Autodesk Fusion 360 part; units mm, degrees
note: some values were not read from the file. Set by a fixed rule: which face or edge a step refers to.
(part 2 of 5)
sketch "Sketch25" plane through (0, 0, 115) normal (0, 0, 1) x (-1, 0, 0)
  line L0 (-26, -108.2203) -> (-26, -178)
  line L1 (-26, -178) -> (-184, -178)
  line L2 (-184, -178) -> (-184, -108.2203)
  line L3 (-184, -108.2203) -> (-180.316, -106.8794)
  arc A0 (-180.316, -106.8794) -> (-179, -105) centre (-181, -105) ccw
  line L4 (-179, -105) -> (-179, -99)
  arc A1 (-179, -99) -> (-180.316, -97.1206) centre (-181, -99) ccw
  line L5 (-180.316, -97.1206) -> (-184, -95.7797)
  line L6 (-184, -95.7797) -> (-184, -56)
  spline S0 degree 3 poles (-184, -56) (-184, -53.3075) (-183.9037, -51.0109) (-183.6552, -49.1696) (-183.4152, -47.3913) (-183.0542, -46.0543) (-182.4179, -44.7239) (-181.7989, -43.4297) (-180.8711, -42.0696) (-179.3518, -40.4458) (-177.5325, -38.5013) (-174.8564, -36.2157) (-171.5158, -33.7703) (-166.6133, -30.1816) (-160.3099, -26.2473) (-154.1768, -22.9953) (-150.0182, -20.7903) (-145.9518, -18.9172) (-142.5291, -17.6934) (-139.736, -16.6948) (-137.3746, -16.1501) (-135.7618, -16.0299) (-135.486, -16.0093) (-135.2319, -16) (-135, -16) knots -1 -1 -1 -1 -0.872949 -0.872949 -0.872949 -0.750244 -0.750244 -0.750244 -0.630875 -0.630875 -0.630875 -0.48793 -0.48793 -0.48793 -0.278155 -0.278155 -0.278155 -0.135918 -0.135918 -0.135918 -0.019847 -0.019847 -0.019847 0 0 0 0
  line L7 (-135, -16) -> (-75, -16)
  spline S1 degree 3 poles (-75, -16) (-73.6407, -16) (-71.4915, -16.3704) (-68.8469, -17.2246) (-63.8244, -18.8468) (-57.0667, -22.1371) (-50.6302, -25.8861) (-45.8029, -28.6979) (-41.1682, -31.7394) (-37.4534, -34.5352) (-34.6662, -36.633) (-32.4058, -38.5922) (-30.788, -40.2974) (-29.2773, -41.8897) (-28.3285, -43.2367) (-27.6926, -44.499) (-27.0341, -45.806) (-26.6597, -47.0839) (-26.4026, -48.7672) (-26.1107, -50.6784) (-26, -53.108) (-26, -56) knots 0 0 0 0 0.116327 0.116327 0.116327 0.337245 0.337245 0.337245 0.502934 0.502934 0.502934 0.627254 0.627254 0.627254 0.743338 0.743338 0.743338 0.863534 0.863534 0.863534 1 1 1 1
  line L8 (-26, -56) -> (-26, -95.7797)
  line L9 (-26, -95.7797) -> (-29.684, -97.1206)
  arc A2 (-29.684, -97.1206) -> (-31, -99) centre (-29, -99) ccw
  line L10 (-31, -99) -> (-31, -105)
  line L11 (-26, -104.5) -> (-28.6, -104.5)
  line L12 (-28.6, -104.5) -> (-28.6, -102)
  line L13 (-29.5, -99.2) -> (-26, -99.2)
  line L14 (-184, -99.2) -> (-180.5, -99.2)
  line L15 (-180.5, -99.2) -> (-180.5, -104.8)
  line L16 (-180.5, -104.8) -> (-184, -104.8)
  line L17 (-30, 0) -> (-180, 0)
  arc A3 (-180, 0) -> (-210, -30) centre (-180, -30) ccw
  line L18 (-210, -30) -> (-210, -180)
  arc A4 (-210, -180) -> (-180, -210) centre (-180, -180) ccw
  line L19 (-180, -210) -> (-30, -210)
  arc A5 (-30, -210) -> (0, -180) centre (-30, -180) ccw
  line L20 (0, -180) -> (0, -30)
  arc A6 (0, -30) -> (-30, 0) centre (-30, -30) ccw
  line L21 (-31, -102) -> (-31, -178)
  line L22 (-31, -102) -> (-31, -30)
  line L23 (-179, -102) -> (-179, -178)
  line L24 (-179, -102) -> (-179, -26)
  line L25 (-26, -99.2) -> (-26, -104.5)
  arc A7 (-31, -105) -> (-29.684, -106.8794) centre (-29, -105) ccw
  line L26 (-29.684, -106.8794) -> (-26, -108.2203)
  circle A8 centre (-199, -108) radius 3.5
  circle A9 centre (-11, -108) radius 3.5
  ellipse E0 centre (-105, -188.2858) end of major axis (-105, -180.5592) minor radius 5.4567
  circle A10 centre (-199, -175) radius 2
  circle A11 centre (-199, -35) radius 2
  circle A12 centre (-11, -35) radius 2
  line L27 (-28.6, -102) -> (-29.5, -102)
  line L28 (-29.5, -102) -> (-29.5, -99.2)
  line L29 (-184, -104.8) -> (-184, -99.2)
  circle A13 centre (-11, -70) radius 2
  circle A14 centre (-199, -70) radius 2
  circle A15 centre (-11, -140) radius 2
  circle A16 centre (-11, -175) radius 2
  circle A17 centre (-199, -140) radius 2
  constraint midpoint L10 L21.start
  constraint coincident L1 L21.end
  constraint perpendicular L1 L21
  constraint parallel L10 L22
  constraint midpoint L4 L23.start
  constraint coincident L1 L23.end
  constraint perpendicular L1 L23
  constraint parallel L4 L24
extrude "Extrude1'" add sketch "Sketch25" along normal blind 10 separate body contours L0 L1 L21 A7 L26 | L1 L2 L3 A0 L23 | S1 L8 L9 A2 L22 | A1 L5 L6 S0 L24 | L11 L12 L13 L25 L27 L28 | L14 L15 L16 L29 | L17 A3 L18 A4 L19 A5 L20 A6 | A8 | A9 makes body 5 in component "inner_adapter"
sketch "Sketch33" plane through (0, 0, 125) normal (0, 0, 1) x (-1, 0, 0)
  line L0 (-179, -178) -> (-179, -40.0766)
  spline S0 degree 3 poles (-179, -40.0766) (-177.1947, -38.2144) (-174.6472, -36.0625) (-171.5158, -33.7703) (-166.6133, -30.1816) (-160.3099, -26.2473) (-154.1768, -22.9953) (-150.0182, -20.7903) (-145.9518, -18.9172) (-142.5291, -17.6934) (-139.736, -16.6948) (-137.3746, -16.1501) (-135.7618, -16.0299) (-135.486, -16.0093) (-135.2319, -16) (-135, -16) knots -0.621923 -0.621923 -0.621923 -0.621923 -0.48793 -0.48793 -0.48793 -0.278155 -0.278155 -0.278155 -0.135918 -0.135918 -0.135918 -0.019847 -0.019847 -0.019847 0 0 0 0
  line L1 (-135, -16) -> (-75, -16)
  spline S1 degree 3 poles (-75, -16) (-73.6407, -16) (-71.4915, -16.3704) (-68.8469, -17.2246) (-63.8244, -18.8468) (-57.0667, -22.1371) (-50.6302, -25.8861) (-45.8029, -28.6979) (-41.1682, -31.7394) (-37.4534, -34.5352) (-34.7859, -36.5429) (-32.601, -38.4237) (-31, -40.0763) knots 0 0 0 0 0.116327 0.116327 0.116327 0.337245 0.337245 0.337245 0.502934 0.502934 0.502934 0.621914 0.621914 0.621914 0.621914
  line L2 (-31, -40.0763) -> (-31, -178)
  line L3 (-31, -178) -> (-179, -178)
  arc A0 (0, -30) -> (-30, 0) centre (-30, -30) ccw
  line L4 (-30, 0) -> (-180, 0)
  arc A1 (-180, 0) -> (-210, -30) centre (-180, -30) ccw
  line L5 (-210, -30) -> (-210, -180)
  arc A2 (-210, -180) -> (-180, -210) centre (-180, -180) ccw
  line L6 (-180, -210) -> (-30, -210)
  arc A3 (-30, -210) -> (0, -180) centre (-30, -180) ccw
  line L7 (0, -180) -> (0, -30)
  line L8 (-109.7559, -178) -> (-100.2441, -178)
  ellipse E0 centre (-105, -188.2858) end of major axis (-105, -180.5592) minor radius 5.4567
  circle A4 centre (-11, -175) radius 2
  circle A5 centre (-199, -175) radius 2
  circle A6 centre (-11, -35) radius 2
  circle A7 centre (-199, -35) radius 2
  circle A8 centre (-199, -35) radius 3.5
  circle A9 centre (-199, -175) radius 3.5
  circle A10 centre (-11, -175) radius 3.5
  circle A11 centre (-11, -35) radius 3.5
  circle A12 centre (-11, -35) radius 2
  ellipse E1 centre (-105, -188.2858) end of major axis (-105, -180.5592) minor radius 5.4567
  circle A13 centre (-199, -175) radius 2
  circle A14 centre (-199, -35) radius 2
  circle A15 centre (-199, -140) radius 2
  circle A16 centre (-11, -140) radius 2
  circle A17 centre (-199, -70) radius 2
  circle A18 centre (-11, -175) radius 2
  circle A19 centre (-11, -70) radius 2
  dimension "d225" = 7
  dimension "d226" = 7
  dimension "d227" = 7
  dimension "d228" = 7
  constraint concentric A7 A8
  constraint concentric A5 A9
  constraint concentric A4 A10
  constraint concentric A6 A11
  measures "d225" diameter of A8
  measures "d226" diameter of A9
  measures "d227" diameter of A10
  measures "d228" diameter of A11
extrude "Extrude5'" cut sketch "Sketch33" against normal blind 5 contours A8 | A9 | A10 | A11 bodies 5 in component "inner_adapter"
sketch "Sketch34" plane through (0, 0, 125) normal (0, 0, 1) x (-1, 0, 0)
  circle A0 centre (-11, -175) radius 3.5
  circle A1 centre (-199, -175) radius 3.5
  circle A2 centre (-11, -35) radius 3.5
  circle A3 centre (-199, -35) radius 3.5
  line L0 (-179, -178) -> (-179, -40.0766)
  spline S0 degree 3 poles (-179, -40.0766) (-177.1947, -38.2144) (-174.6472, -36.0625) (-171.5158, -33.7703) (-166.6133, -30.1816) (-160.3099, -26.2473) (-154.1768, -22.9953) (-150.0182, -20.7903) (-145.9518, -18.9172) (-142.5291, -17.6934) (-139.736, -16.6948) (-137.3746, -16.1501) (-135.7618, -16.0299) (-135.486, -16.0093) (-135.2319, -16) (-135, -16) knots -0.621923 -0.621923 -0.621923 -0.621923 -0.48793 -0.48793 -0.48793 -0.278155 -0.278155 -0.278155 -0.135918 -0.135918 -0.135918 -0.019847 -0.019847 -0.019847 0 0 0 0
  line L1 (-135, -16) -> (-75, -16)
  spline S1 degree 3 poles (-75, -16) (-73.6407, -16) (-71.4915, -16.3704) (-68.8469, -17.2246) (-63.8244, -18.8468) (-57.0667, -22.1371) (-50.6302, -25.8861) (-45.8029, -28.6979) (-41.1682, -31.7394) (-37.4534, -34.5352) (-34.7859, -36.5429) (-32.601, -38.4237) (-31, -40.0763) knots 0 0 0 0 0.116327 0.116327 0.116327 0.337245 0.337245 0.337245 0.502934 0.502934 0.502934 0.621914 0.621914 0.621914 0.621914
  line L2 (-31, -40.0763) -> (-31, -178)
  line L3 (-31, -178) -> (-179, -178)
  arc A4 (0, -30) -> (-30, 0) centre (-30, -30) ccw
  line L4 (-30, 0) -> (-180, 0)
  arc A5 (-180, 0) -> (-210, -30) centre (-180, -30) ccw
  line L5 (-210, -30) -> (-210, -180)
  arc A6 (-210, -180) -> (-180, -210) centre (-180, -180) ccw
  line L6 (-180, -210) -> (-30, -210)
  arc A7 (-30, -210) -> (0, -180) centre (-30, -180) ccw
  line L7 (0, -180) -> (0, -30)
  circle A8 centre (-11, -175) radius 3.5
  circle A9 centre (-199, -175) radius 3.5
  circle A10 centre (-11, -35) radius 3.5
  circle A11 centre (-199, -35) radius 3.5
  line L8 (-179, -178) -> (-179, -40.0766)
  spline S2 degree 3 poles (-179, -40.0766) (-177.1947, -38.2144) (-174.6472, -36.0625) (-171.5158, -33.7703) (-166.6133, -30.1816) (-160.3099, -26.2473) (-154.1768, -22.9953) (-150.0182, -20.7903) (-145.9518, -18.9172) (-142.5291, -17.6934) (-139.736, -16.6948) (-137.3746, -16.1501) (-135.7618, -16.0299) (-135.486, -16.0093) (-135.2319, -16) (-135, -16) knots -0.621923 -0.621923 -0.621923 -0.621923 -0.48793 -0.48793 -0.48793 -0.278155 -0.278155 -0.278155 -0.135918 -0.135918 -0.135918 -0.019847 -0.019847 -0.019847 0 0 0 0
  line L9 (-135, -16) -> (-75, -16)
  spline S3 degree 3 poles (-75, -16) (-73.6407, -16) (-71.4915, -16.3704) (-68.8469, -17.2246) (-63.8244, -18.8468) (-57.0667, -22.1371) (-50.6302, -25.8861) (-45.8029, -28.6979) (-41.1682, -31.7394) (-37.4534, -34.5352) (-34.7859, -36.5429) (-32.601, -38.4237) (-31, -40.0763) knots 0 0 0 0 0.116327 0.116327 0.116327 0.337245 0.337245 0.337245 0.502934 0.502934 0.502934 0.621914 0.621914 0.621914 0.621914
  line L10 (-31, -40.0763) -> (-31, -178)
  line L11 (-31, -178) -> (-179, -178)
  arc A12 (0, -30) -> (-30, 0) centre (-30, -30) ccw
  line L12 (-30, 0) -> (-180, 0)
  arc A13 (-180, 0) -> (-210, -30) centre (-180, -30) ccw
  line L13 (-210, -30) -> (-210, -180)
  arc A14 (-210, -180) -> (-180, -210) centre (-180, -180) ccw
  line L14 (-180, -210) -> (-30, -210)
  arc A15 (-30, -210) -> (0, -180) centre (-30, -180) ccw
  line L15 (0, -180) -> (0, -30)
  line L16 (-179.0609, -163) -> (-179, -173)
  line L17 (-184, -183) -> (-184, -38.0508)
  spline S4 degree 3 poles (-184, -38.0508) (-183.53, -37.5659) (-183.0599, -37.0811) (-182.5899, -36.5963) (-180.4883, -34.4285) (-177.7611, -32.1455) (-174.4691, -29.7357) (-169.3238, -25.9693) (-162.8741, -21.9475) (-156.519, -18.5779) (-152.2041, -16.29) (-147.9761, -14.3309) (-144.2124, -12.9853) (-141.9329, -12.1703) (-139.8769, -11.6068) (-138.0391, -11.287) (-137.3844, -11.1731) (-136.7557, -11.0901) (-136.1336, -11.0437) (-135.7424, -11.0145) (-135.3658, -11) (-135, -11) knots -0.65681 -0.65681 -0.65681 -0.65681 -0.621923 -0.621923 -0.621923 -0.48793 -0.48793 -0.48793 -0.278155 -0.278155 -0.278155 -0.135918 -0.135918 -0.135918 -0.050335 -0.050335 -0.050335 -0.019847 -0.019847 -0.019847 0 0 0 0
  line L18 (-135, -11) -> (-75, -11)
  spline S5 degree 3 poles (-75, -11) (-73.6669, -11) (-72.3215, -11.1868) (-70.7827, -11.5209) (-69.7039, -11.7551) (-68.5449, -12.0678) (-67.3101, -12.4666) (-63.5716, -13.6741) (-59.3264, -15.5672) (-54.921, -17.8316) (-52.6617, -18.993) (-50.3688, -20.252) (-48.1137, -21.5656) (-43.134, -24.4661) (-38.3659, -27.5905) (-34.4467, -30.5403) (-31.6285, -32.6614) (-29.2725, -34.6734) (-27.4088, -36.5974) (-26.9392, -37.0821) (-26.4696, -37.5669) (-26, -38.0516) knots 0 0 0 0 0.068385 0.068385 0.068385 0.116327 0.116327 0.116327 0.262353 0.262353 0.262353 0.337245 0.337245 0.337245 0.502934 0.502934 0.502934 0.621914 0.621914 0.621914 0.656812 0.656812 0.656812 0.656812
  line L19 (-26, -38.0516) -> (-26, -183)
  line L20 (-26, -183) -> (-184, -183)
  line L21 (-135, -17) -> (-75, -17)
  spline S6 degree 3 poles (-75, -17) (-73.8223, -17) (-71.7285, -17.3447) (-69.1542, -18.1762) (-64.2585, -19.7574) (-57.5268, -23.0263) (-51.1335, -26.7502) (-46.3366, -29.5442) (-41.7286, -32.5691) (-38.0548, -35.3342) (-35.5737, -37.2016) (-33.5233, -38.9532) (-32, -40.4851) knots 0 0 0 0 0.116327 0.116327 0.116327 0.337245 0.337245 0.337245 0.502934 0.502934 0.502934 0.61486 0.61486 0.61486 0.61486
  line L22 (-32, -40.4851) -> (-32, -177)
  line L23 (-32, -177) -> (-178, -177)
  line L24 (-178, -177) -> (-178, -40.4855)
  spline S7 degree 3 poles (-178, -40.4855) (-176.2702, -38.7472) (-173.8613, -36.7265) (-170.9251, -34.5772) (-166.0712, -31.0241) (-159.7971, -27.1072) (-153.7083, -23.8788) (-149.581, -21.6904) (-145.547, -19.8344) (-142.1924, -18.6351) (-139.459, -17.6578) (-137.1491, -17.1361) (-135.6875, -17.0271) (-135.4348, -17.0083) (-135.2051, -17) (-135, -17) knots -0.614871 -0.614871 -0.614871 -0.614871 -0.48793 -0.48793 -0.48793 -0.278155 -0.278155 -0.278155 -0.135918 -0.135918 -0.135918 -0.019847 -0.019847 -0.019847 0 0 0 0
  ellipse E0 centre (-105, -188.2858) end of major axis (-105, -180.5592) minor radius 5.4567
  ellipse E1 centre (-105, -188.2858) end of major axis (-105, -180.5592) minor radius 5.4567
  circle A16 centre (-199, -140) radius 2
  circle A17 centre (-11, -140) radius 2
  circle A18 centre (-199, -70) radius 2
  circle A19 centre (-11, -70) radius 2
  circle A20 centre (-199, -140) radius 2
  circle A21 centre (-11, -140) radius 2
  circle A22 centre (-199, -70) radius 2
  circle A23 centre (-11, -70) radius 2
  dimension "d234" = -5
  dimension "d235" = 1
  constraint coincident L8 L16.end
extrude "Extrude6'" add sketch "Sketch34" along normal blind 80 contours L17 S4 L18 S5 L19 L20 E0 E1 | L20 E0 E1 picked at (-103.7762, -182.6498) bodies 5 in component "inner_adapter"
ref_plane "WorkPlane5" through (184, 102, 115) normal (0.422618, 0, 0.906308) x (0, -1, 0)
sketch "Sketch35" plane through (184, 102, 115) normal (0.422618, 0, 0.906308) x (0, -1, 0)
  line L0 (-2.8, -3.1721) -> (-2.8, 0)
  line L1 (-2.8, -3.1721) -> (2.8, -3.1721)
  line L2 (2.8, -3.1721) -> (2.8, 0)
  line L3 (-2.8, 0) -> (2.8, 0)
extrude "Extrude7" cut sketch "Sketch35" along normal blind 15 and the other way blind 2 bodies 5 in component "inner_adapter"
ref_plane "WorkPlane6" through (105, 109.0383, 160) normal (-1, 0, 0) x (0, -1, 0)
mirror "Mirror1" about plane through (105, 109.0383, 160) normal (-1, 0, 0) of "Extrude7" in component "inner_adapter"
sketch "Sketch36" plane through (179, 0, 0) normal (-1, 0, 0) x (0, -1, 0)
  line L0 (-178, 115) -> (-40.0766, 115)
  line L1 (-40.0766, 115) -> (-40.0766, 205)
  line L2 (-40.0766, 205) -> (-178, 205)
  line L3 (-178, 205) -> (-178, 115)
  circle A0 centre (-173, 130) radius 3.5
  line L4 (-173, 130) -> (-176.5, 130)
  line L5 (-176.5, 130) -> (-176.5, 205)
  line L6 (-176.5, 205) -> (-173, 205)
  line L7 (-173, 130) -> (-169.5, 130)
  line L8 (-169.5, 130) -> (-169.5, 205)
  line L9 (-169.5, 205) -> (-173, 205)
  line L10 (-173, 205) -> (-173, 130)
  line L11 (-171.5, 133.1623) -> (-171.5, 205)
  line L12 (-180, 125) -> (-30, 125)
  dimension "d245" = 7
  dimension "d246" = 5
  dimension "d247" = 3.5
  dimension "d248" = 3.5
  dimension "d267" = 5
  dimension "d412" = 5
  constraint horizontal L4
  constraint vertical L5
  constraint horizontal L6
  constraint coincident L2 L5.end
  constraint coincident A0.centre L4.start
  constraint horizontal L7
  constraint vertical L8
  constraint horizontal L9
  constraint vertical L10
  constraint coincident L2 L8.end
  constraint coincident A0 L11.start
  constraint coincident L2 L11.end
  constraint perpendicular L2 L11
  measures "d245" diameter of A0
  measures "d246" distance of L3 A0.centre
  measures "d247" distance of A0.centre L4.end
  measures "d248" distance of A0.centre L7.end
  measures "d267" distance of L5 L11
  measures "d412" distance of L4 L12
extrude "Extrude8'" cut sketch "Sketch36" against normal blind 5 contours L2 A0 L5 L6 L10 | L2 A0 L9 L10 L11 | A0 L4 L7 | A0 L4 L10 | A0 L7 L10 bodies 5 in component "inner_adapter"
mirror "Mirror2" about plane through (105, 109.0383, 160) normal (-1, 0, 0) of "Extrude8'" in component "inner_adapter"
ref_plane "WorkPlane7" through (180.7273, 173, 126.5) normal (0, 0, 1) x (0, 1, 0)
sketch "Sketch38" plane through (180.1788, 173, 126.5) normal (0, 0, 1) x (1, 0, 0)
  line L0 (-1.1788, 3.5) -> (3.8212, 3.5)
  line L1 (-1.1788, 3) -> (3.8212, 3)
  line L2 (-1.1788, 3) -> (-2.1788, 3)
  spline S0 degree 3 poles (-1.1788, -132.9234) (-2.9841, -134.7856) (-5.5316, -136.9375) (-8.663, -139.2297) (-13.5655, -142.8184) (-19.8689, -146.7527) (-26.0021, -150.0047) (-30.1606, -152.2097) (-34.227, -154.0828) (-37.6497, -155.3066) (-40.4428, -156.3052) (-42.8042, -156.8499) (-44.417, -156.9701) (-44.6928, -156.9907) (-44.9469, -157) (-45.1788, -157) knots -0.621923 -0.621923 -0.621923 -0.621923 -0.48793 -0.48793 -0.48793 -0.278155 -0.278155 -0.278155 -0.135918 -0.135918 -0.135918 -0.019847 -0.019847 -0.019847 0 0 0 0
  line L3 (-45.1788, -157) -> (-105.1788, -157)
  spline S1 degree 3 poles (-105.1788, -157) (-106.5381, -157) (-108.6873, -156.6296) (-111.332, -155.7754) (-116.3544, -154.1532) (-123.1121, -150.8629) (-129.5486, -147.1139) (-134.376, -144.3021) (-139.0107, -141.2606) (-142.7254, -138.4648) (-145.3929, -136.4571) (-147.5779, -134.5763) (-149.1788, -132.9237) knots 0 0 0 0 0.116327 0.116327 0.116327 0.337245 0.337245 0.337245 0.502934 0.502934 0.502934 0.621914 0.621914 0.621914 0.621914
  line L4 (3.8212, -1.4285) -> (3.8212, 3)
  line L5 (-149.1788, -132.9237) -> (-149.1788, -1.5)
  line L6 (-1.1788, -1.5) -> (-1.1788, -132.9234)
  line L7 (-1.1788, 5) -> (-1.1788, 3.5)
  line L8 (3.8212, 3.5) -> (3.8212, -3.5)
  line L9 (-2.1774, 2.972) -> (-2.1774, 3.972)
  line L10 (-2.1788, -1.5) -> (-2.1788, -132.5145)
  spline S2 degree 3 poles (-2.1788, -132.5145) (-3.9086, -134.2528) (-6.3175, -136.2735) (-9.2537, -138.4228) (-14.1076, -141.9759) (-20.3818, -145.8928) (-26.4705, -149.1212) (-30.5978, -151.3096) (-34.6319, -153.1656) (-37.9864, -154.3649) (-40.7198, -155.3422) (-43.0297, -155.8639) (-44.4914, -155.9729) (-44.7441, -155.9917) (-44.9737, -156) (-45.1788, -156) knots -0.614871 -0.614871 -0.614871 -0.614871 -0.48793 -0.48793 -0.48793 -0.278155 -0.278155 -0.278155 -0.135918 -0.135918 -0.135918 -0.019847 -0.019847 -0.019847 0 0 0 0
  line L11 (-45.1788, -156) -> (-105.1788, -156)
  spline S3 degree 3 poles (-105.1788, -156) (-106.3565, -156) (-108.4503, -155.6553) (-111.0246, -154.8238) (-115.9203, -153.2426) (-122.652, -149.9737) (-129.0453, -146.2498) (-133.8422, -143.4558) (-138.4502, -140.4309) (-142.1241, -137.6658) (-144.6051, -135.7984) (-146.6556, -134.0468) (-148.1788, -132.5149) knots 0 0 0 0 0.116327 0.116327 0.116327 0.337245 0.337245 0.337245 0.502934 0.502934 0.502934 0.61486 0.61486 0.61486 0.61486
  line L12 (-148.1788, -132.5149) -> (-148.1788, -1.5)
  line L13 (-148.1788, -1.5) -> (-148.1788, 3.972)
  line L14 (-2.1788, -1.5) -> (-2.1774, 3.972)
  line L15 (-2.18, -2) -> (3.8212, -2)
  line L16 (3.8212, -2) -> (3.8212, 3)
  line L17 (3.8212, 3) -> (-2.18, 3)
  line L18 (-2.18, 3) -> (-2.18, -2)
  line L19 (-2.1774, 3.972) -> (-148.1788, 3.972)
  line L20 (-75.1788, 18.1402) -> (-75.1788, -146.0636)
  line L21 (-154.1788, 3) -> (-148.1776, 3)
  line L22 (-154.1788, -1.4285) -> (-154.1788, 3)
  line L23 (-148.1776, -2) -> (-154.1788, -2)
  line L24 (-148.1776, 3) -> (-148.1776, -2)
  line L25 (-154.1788, 3) -> (-148.1776, 3)
  line L26 (-148.1776, 3) -> (-148.1776, -2)
  line L27 (-148.1776, -2) -> (-154.1788, -2)
  line L28 (-154.1788, -2) -> (-154.1788, 3)
  spline S4 degree 3 poles (-2.6148, -131.5313) (-4.3015, -133.2712) (-6.7772, -135.3707) (-9.8444, -137.6159) (-14.6497, -141.1334) (-20.8946, -145.0328) (-26.939, -148.2377) (-31.035, -150.4095) (-35.0367, -152.2483) (-38.3231, -153.4233) (-40.802, -154.3096) (-42.9157, -154.8054) (-44.2634, -154.9482) (-44.3693, -154.9594) (-44.4702, -154.9685) (-44.5657, -154.9757) (-44.7953, -154.9928) (-45.0005, -155) (-45.1788, -155) knots -0.621923 -0.621923 -0.621923 -0.621923 -0.48793 -0.48793 -0.48793 -0.278155 -0.278155 -0.278155 -0.135918 -0.135918 -0.135918 -0.028304 -0.028304 -0.028304 -0.019847 -0.019847 -0.019847 0 0 0 0
  line L29 (-45.1788, -155) -> (-105.1788, -155)
  spline S5 degree 3 poles (-105.1788, -155) (-105.9646, -155) (-107.4138, -154.8062) (-109.204, -154.3221) (-109.6831, -154.1926) (-110.1886, -154.043) (-110.7173, -153.8722) (-115.0849, -152.4615) (-121.0823, -149.6189) (-126.9331, -146.3093) (-127.4708, -146.0051) (-128.0075, -145.697) (-128.542, -145.3857) (-133.3084, -142.6094) (-137.8898, -139.6011) (-141.5227, -136.8668) (-144.13, -134.9044) (-146.2465, -133.0763) (-147.7423, -131.5321) knots 0 0 0 0 0.091769 0.091769 0.091769 0.116327 0.116327 0.116327 0.318651 0.318651 0.318651 0.337245 0.337245 0.337245 0.502934 0.502934 0.502934 0.621914 0.621914 0.621914 0.621914
  line L30 (-2.6148, -131.5313) -> (-2.1788, -131.0816)
  line L31 (-147.7423, -131.5321) -> (-148.1788, -131.0815)
  dimension "d252" = 0.5
  dimension "d254" = 1
  dimension "d776" = 1
  dimension "d781" = 5
  dimension "d947" = 2
  constraint parallel L1 L2
  constraint perpendicular L1 L4
  constraint vertical L9
  constraint parallel L12 L13
  constraint horizontal L15
  constraint vertical L16
  constraint horizontal L17
  constraint vertical L18
  constraint perpendicular L9 L19
  constraint symmetric L1.end L20 L21.start
  constraint symmetric L4.start L20 L22.start
  constraint symmetric L15.start L20 L23.start
  constraint symmetric L15.end L20 L23.end
  constraint symmetric L17.end L20 L21.end
  constraint horizontal L25
  constraint vertical L26
  constraint horizontal L27
  constraint vertical L28
  constraint coincident L10 L30.end
  constraint coincident L12 L31.end
  measures "d254" distance of L1.start L2.end
  measures "d781" distance of L15.start L17.end
extrude "Extrude1''" add sketch "Sketch38" along normal blind 5 from surface at 1 separate body contours L1 L2 L4 L8 L9 L10 L14 L15 L16 L17 L18 | L9 L10 L12 L13 L14 L18 L19 L24 L26 S4 L29 S5 L30 L31 | L12 L13 L21 L22 L23 L24 L25 L26 L27 L28 makes body 6 in component "Flap"
sketch "Sketch39" plane through (184, 0, 0) normal (-1, 0, 0) x (0, -1, 0)
  line L0 (-171, 127.5) -> (-176, 127.5)
  line L1 (-176, 127.5) -> (-176, 132.5)
  line L2 (-176, 132.5) -> (-171, 132.5)
  line L3 (-171, 132.5) -> (-171, 127.5)
  line L4 (-171, 127.5) -> (-176, 127.5)
  line L5 (-176, 127.5) -> (-176, 132.5)
  line L6 (-176, 132.5) -> (-171, 132.5)
  line L7 (-171, 132.5) -> (-171, 127.5)
  line L8 (-176, 130) -> (-171, 130)
  line L9 (-173.5, 127.5) -> (-173.5, 130)
  circle A0 centre (-173.5, 130) radius 2.55
  dimension "d783" = 5.1
  constraint midpoint L1 L8.start
  constraint perpendicular L1 L8
  constraint midpoint L0 L9.start
  constraint midpoint L8 L9.end
  constraint coincident L9.end A0.centre
  measures "d783" diameter of A0
extrude "Extrude6''" cut sketch "Sketch39" along normal blind 6 contours L0 L3 L4 L7 A0 | L0 L1 L4 L5 A0 | L2 L3 L6 L7 A0 | L1 L2 L5 L6 A0 bodies 6 in component "Flap"
mirror "Mirror4" about plane through (105, 109.0383, 160) normal (-1, 0, 0) of "Extrude6''" in component "Flap"
extrude "Extrude3'" add sketch "Sketch39" against normal blind 5 draft 20 contours L0 L3 L4 L7 L8 L9 A0 | L0 L1 L4 L5 L8 L9 A0 | L1 L2 L3 L5 L6 L7 L8 A0 bodies 6 in component "Flap"
sketch "Sketch41" plane through (189, 0, 0) normal (1, 0, 0) x (0, -1, 0)
  line L0 (-177.8199, -129.3408) -> (-177.8199, -130.6592)
  arc A0 (-177.8199, -130.6592) -> (-174.1592, -134.3199) centre (-173.5, -130) ccw
  line L1 (-174.1592, -134.3199) -> (-172.8408, -134.3199)
  arc A1 (-172.8408, -134.3199) -> (-169.1801, -130.6591) centre (-173.5, -130) ccw
  line L2 (-169.1801, -130.6591) -> (-169.1801, -129.3409)
  arc A2 (-169.1801, -129.3409) -> (-172.8408, -125.6801) centre (-173.5, -130) ccw
  line L3 (-172.8408, -125.6801) -> (-174.1592, -125.6801)
  arc A3 (-174.1592, -125.6801) -> (-177.8199, -129.3408) centre (-173.5, -130) ccw
  line L4 (-173.5, -130) -> (-175.5, -130)
  line L5 (-175.5, -130) -> (-173.5, -130)
  line L6 (-173.5, -130) -> (-171.5, -130)
  line L7 (-175.5, -130) -> (-171.5, -130)
  line L8 (-171.5, -130) -> (-171.5, -140)
  line L9 (-171.5, -140) -> (-175.5, -140)
  line L10 (-175.5, -140) -> (-175.5, -130)
  circle A4 centre (-173.5, -130) radius 10
  constraint coincident A0.centre A1.centre
  constraint horizontal L4
  constraint parallel L4 L6
  constraint horizontal L7
  constraint vertical L8
  constraint horizontal L9
  constraint vertical L10
extrude "Extrude7'" add sketch "Sketch41" along normal blind 2 contours L0 A0 A1 L2 A2 L3 A3 L4 L5 L6 L7 L8 L10 | L0 A0 A1 L2 A2 L3 A3 L8 L10 A4 | A0 L1 A1 L4 L5 L6 L7 L8 L10 | A0 L1 A1 L8 L10 A4 bodies 6 in component "Flap"
mirror "Mirror3" about plane through (105, 109.0383, 160) normal (-1, 0, 0) of "Extrude3'", "Extrude7'" in component "Flap"
sketch "Sketch42" plane through (0, 0, 125) normal (0, 0, 1) x (-1, 0, 0)
  line L0 (-19, -163.5) -> (-18.9999, -163.5)
  line L1 (-21, -183.5) -> (-21, -163.5)
  line L2 (-19, -163.5) -> (-19, -183.5)
  line L3 (-21, -163.5) -> (-21, -183.5)
  line L4 (-18, -160.5) -> (-18, -186.5)
  line L5 (-18, -186.5) -> (-25, -186.5)
  line L6 (-25, -186.5) -> (-25, -160.5)
  line L7 (-25, -160.5) -> (-18, -160.5)
  line L8 (-21, -163.5) -> (-21, -183.5)
  dimension "d818" = 3
  dimension "d819" = 7
  dimension "d820" = 3
  dimension "d821" = 3
  constraint coincident L0.start L2.start
  constraint coincident L1.start L3.end
  constraint coincident L1.end L3.start
  constraint vertical L4
  constraint horizontal L5
  constraint vertical L6
  constraint perpendicular L4 L7
  measures "d818" distance of L4 L8
  measures "d819" distance of L6.end L4.start
  measures "d820" distance of L0.start L7
  measures "d821" distance of L2.end L5
extrude "Extrude9" cut sketch "Sketch42" against normal blind 7 bodies 5 in component "inner_adapter"
mirror "Mirror3'" about plane through (105, 109.0383, 160) normal (-1, 0, 0) of "Extrude9" in component "inner_adapter"
sketch "Sketch90" plane through (0, 183, 0) normal (0, 1, 0) x (-1, 0, 0)
  line L0 (-184, 125) -> (-108.98, 125)
  line L1 (-108.98, 125) -> (-108.98, 185)
  line L2 (-108.98, 185) -> (-184, 185)
  line L3 (-184, 185) -> (-184, 125)
  line L4 (-179, 130) -> (-179, 185)
  line L5 (-21, 145) -> (-21, 140)
  circle A0 centre (-181.4998, 134.998) radius 1.9
  line L6 (-181.5, 129.998) -> (-181.4998, 134.998)
  line L7 (-26, 127.5) -> (-21, 125.6801)
  line L8 (-26, 132.5) -> (-21, 134.3199)
  line L9 (-184, 127.5) -> (-189, 125.6801)
  line L10 (-184, 132.5) -> (-189, 134.3199)
  line L11 (-26, 132.5) -> (-32, 132.5)
  line L12 (-32, 127.5) -> (-26, 127.5)
  line L13 (-178, 132.5) -> (-184, 132.5)
  line L14 (-184, 127.5) -> (-178, 127.5)
  line L15 (-189, 140) -> (-189, 134.3199)
  line L16 (-189, 125.6801) -> (-189, 120)
  line L17 (-191, 140) -> (-191, 120)
  line L18 (-189, 140) -> (-191, 140)
  line L19 (-189, 120) -> (-191, 120)
  line L20 (-21, 140) -> (-21, 134.3199)
  line L21 (-21, 125.6801) -> (-21, 120)
  line L22 (-19, 140) -> (-19, 120)
  line L23 (-19, 140) -> (-21, 140)
  line L24 (-19, 120) -> (-21, 120)
  line L25 (-32, 132.5) -> (-32.4365, 132.5)
  line L26 (-32.4365, 132.5) -> (-75, 132.5)
  line L27 (-75, 132.5) -> (-135, 132.5)
  line L28 (-135, 132.5) -> (-177.564, 132.5)
  line L29 (-177.564, 132.5) -> (-178, 132.5)
  line L30 (-177.564, 127.5) -> (-178, 127.5)
  line L31 (-177.564, 127.5) -> (-135, 127.5)
  line L32 (-135, 127.5) -> (-75, 127.5)
  line L33 (-75, 127.5) -> (-32.4365, 127.5)
  line L34 (-32.4365, 127.5) -> (-32, 127.5)
  line L35 (-101.02, 125) -> (-26, 125)
  line L36 (-26, 125) -> (-26, 205)
  line L37 (-26, 205) -> (-184, 205)
  line L38 (-184, 205) -> (-184, 125)
  line L39 (-184, 125) -> (-108.98, 125)
  line L40 (-108.98, 125) -> (-101.02, 125)
  dimension "d770" = 3.8
  dimension "d771" = 5
  constraint coincident A0.centre L6.end
  measures "d770" diameter of A0
  measures "d771" distance of L6.start A0.centre
extrude "Extrude54" cut sketch "Sketch90" against normal blind 20 contours A0 bodies 5 in component "inner_adapter"
mirror "Mirror7" about plane through (105, 109.0383, 160) normal (-1, 0, 0) of "Extrude54" in component "inner_adapter"
sketch "Sketch91" plane through (19, 0, 0) normal (-1, 0, 0) x (0, -1, 0)
  circle A0 centre (-173.5, 130) radius 10
sketch "Sketch92" plane through (19, 0, 0) normal (1, 0, 0) x (0, 1, 0)
  line L0 (186.5, 125) -> (186.5, 118)
  line L1 (160.5, 118) -> (186.5, 118)
  line L2 (160.5, 125) -> (160.5, 118)
  line L3 (160.5, 126.75) -> (160.5, 133.25)
  line L4 (160.5, 133.25) -> (166.5, 133.25)
  line L5 (173.5, 130) -> (160.5, 130)
  line L6 (160.5, 133.25) -> (157.5, 133.25)
  line L7 (160.5, 126.75) -> (157.5, 126.75)
  line L8 (157.5, 126.75) -> (157.5, 133.25)
  line L9 (157.5, 133.25) -> (160.5, 133.25)
  line L10 (160.5, 133.25) -> (160.5, 126.75)
  line L11 (166.5, 133.25) -> (168, 133.25)
  line L12 (166.5, 133.25) -> (166.5, 130)
  line L13 (168, 133.25) -> (160.5, 133.25)
  line L14 (160.5, 133.25) -> (160.5, 126.75)
  line L15 (160.5, 126.75) -> (168, 126.75)
  line L16 (168, 126.75) -> (168, 133.25)
  line L17 (166.5, 130) -> (165, 130)
  circle A0 centre (173.5, 130) radius 8.5
  line L18 (166.5, 130) -> (168, 130)
  circle A1 centre (173.5, 130) radius 5.5
  line L19 (173.5, 130) -> (166.4289, 122.9289)
  line L20 (173.5, 130) -> (180.5711, 122.9289)
  line L21 (160.5, 125) -> (157.5, 125)
  line L22 (157.5, 125) -> (157.5, 127)
  line L23 (157.5, 127) -> (160.5, 127)
  line L24 (160.5, 127) -> (160.5, 125)
  line L25 (160.5, 135.25) -> (160.5, 133.25)
  line L26 (157.5, 133.25) -> (157.5, 126.75)
  circle A2 centre (173.5, 130) radius 10
  line L27 (160.5, 135.25) -> (157.5, 135.25)
  line L28 (157.5, 135.25) -> (157.5, 133.25)
  line L29 (157.5, 133.25) -> (160.5, 133.25)
  line L30 (160.5, 133.25) -> (160.5, 135.25)
  line L31 (160.5, 135.25) -> (162.5, 135.25)
  line L32 (162.5, 135.25) -> (162.5, 133.25)
  line L33 (162.5, 133.25) -> (160.5, 133.25)
  line L34 (160.5, 133.25) -> (160.5, 135.25)
  line L35 (160.5, 125) -> (162.5, 125)
  line L36 (162.5, 125) -> (162.5, 126.75)
  line L37 (162.5, 126.75) -> (160.5, 126.75)
  line L38 (160.5, 126.75) -> (160.5, 125)
  line L39 (162.5, 133.25) -> (162.5, 126.75)
  dimension "d822" = 6.5
  dimension "d823" = 6
  dimension "d824" = 3
  dimension "d825" = 1.5
  dimension "d826" = 1.5
  dimension "d827" = 1.5
  dimension "d828" = 10
  dimension "d829" = 45
  dimension "d830" = 10
  dimension "d831" = 90
  dimension "d832" = 2
  dimension "d834" = 13
  dimension "d1054" = 2
  dimension "d1055" = 2
  constraint parallel L2 L3
  constraint perpendicular L2 L4
  constraint coincident L3 L5.end
  constraint perpendicular L3 L5
  constraint midpoint L3 L5.end
  constraint perpendicular L3 L6
  constraint horizontal L7
  constraint vertical L8
  constraint horizontal L9
  constraint vertical L10
  constraint horizontal L11
  constraint coincident L5 L12.end
  constraint perpendicular L5 L12
  constraint horizontal L13
  constraint vertical L14
  constraint horizontal L15
  constraint vertical L16
  constraint perpendicular L12 L17
  constraint coincident L5.start A0.centre
  constraint coincident L17.end A0
  constraint perpendicular L16 L18
  constraint concentric A0 A1
  constraint coincident L18.end A1
  constraint horizontal L21
  constraint vertical L22
  constraint horizontal L23
  constraint vertical L24
  constraint coincident L2.start L21.start
  constraint vertical L25
  constraint collinear L2 L14
  constraint vertical L26
  constraint collinear L8 L22
  constraint horizontal L27
  constraint vertical L28
  constraint horizontal L29
  constraint vertical L30
  constraint horizontal L31
  constraint vertical L32
  constraint horizontal L33
  constraint vertical L34
  constraint horizontal L35
  constraint vertical L36
  constraint horizontal L37
  constraint vertical L38
  constraint perpendicular L15 L39
  measures "d822" distance of L3.start L3.end
  measures "d823" distance of L3.end L4.end
  measures "d824" distance of L3.end L6.end
  measures "d825" distance of L4.end L11.end
  measures "d826" distance of L12.end L17.end
  measures "d827" distance of L12.end L18.end
  measures "d828" distance of L5.start L19.end
  measures "d829" angle of L5 L19
  measures "d830" distance of L5.start L20.end
  measures "d831" angle of L19 L20
  measures "d832" distance of L3.end L25.start
  measures "d834" distance of L5.start L5.end
  measures "d1054" distance of L25.start L31.end
  measures "d1055" distance of L2.start L35.end
extrude "Extrude8''" cut sketch "Sketch92" along normal blind 2 contours A0 A1 L19 L20 bodies 6 in component "Flap"
sketch "Sketch93" plane through (191, 0, 0) normal (1, 0, 0) x (0, 1, 0)
  circle A0 centre (173.5, 130) radius 10
  circle A1 centre (173.5, 130) radius 8.5
  circle A2 centre (173.5, 130) radius 5.5
  line L0 (173.5, 130) -> (180.5711, 137.0711)
  line L1 (173.5, 130) -> (185, 130)
  line L2 (173.5, 130) -> (166.4289, 137.0711)
  dimension "d853" = 17
  dimension "d854" = 11
  dimension "d855" = 10
  dimension "d856" = 45
  dimension "d857" = 10
  dimension "d858" = 90
  constraint concentric A0 A1
  constraint concentric A0 A2
  constraint coincident A0.centre A1.centre
  constraint horizontal L1
  measures "d853" diameter of A1
  measures "d854" diameter of A2
  measures "d855" distance of A0.centre L0.end
  measures "d856" angle of L0 L1
  measures "d857" distance of A0.centre L2.end
  measures "d858" angle of L0 L2
extrude "Extrude9'" cut sketch "Sketch93" against normal blind 2 contours A1 A2 L0 L2 bodies 6 in component "Flap"
sketch "Sketch108" plane through (0, 183, 0) normal (0, 1, 0) x (-1, 0, 0)
  line L0 (-182.5, 180) -> (-184, 180)
  line L1 (-184, 125) -> (-108.98, 125)
  line L2 (-26, 125) -> (-26, 185)
  line L3 (-26, 185) -> (-182.5, 185)
  circle A0 centre (-28.5002, 134.998) radius 1.9
  line L4 (-108.98, 125) -> (-108.98, 180)
  line L5 (-105, 180.0157) -> (-105, 175.0157)
  line L6 (-105, 175.0157) -> (-105, 170.0157)
  circle A1 centre (-105, 170.0157) radius 5.25
  line L7 (-184, 180) -> (-184, 125)
  line L8 (-108.98, 125) -> (-101.02, 125)
  line L9 (-101.02, 125) -> (-26, 125)
  line L10 (-182.5, 185) -> (-182.5, 180)
  circle A2 centre (-181.4998, 134.998) radius 1.9
  line L11 (-184, 205) -> (-184, 125)
  line L12 (-184, 125) -> (-108.98, 125)
  line L13 (-108.98, 125) -> (-101.02, 125)
  line L14 (-101.02, 125) -> (-26, 125)
  line L15 (-26, 125) -> (-26, 205)
  line L16 (-26, 205) -> (-184, 205)
  circle A3 centre (-28.5002, 134.998) radius 1.9
  circle A4 centre (-181.4998, 134.998) radius 1.9
  line L17 (-101.02, 125) -> (-101.02, 180.0315)
  line L18 (-108.98, 180) -> (-101.02, 180.0315)
  point P0 (-105, 180.0157)
  dimension "d980" = 5
  dimension "d981" = 5
  dimension "d982" = 10.5
  constraint parallel L5 L6
  constraint coincident L6.end A1.centre
  constraint coincident L8.end L9.start
  constraint perpendicular L14 L17
  constraint midpoint L18 P0
  constraint coincident P0 L5.start
  constraint parallel L4 L5
  measures "d980" distance of P0 L5.end
  measures "d981" distance of L5.end L6.end
  measures "d982" diameter of A1
extrude "Extrude63" cut sketch "Sketch108" against normal blind 6 contours L4 A1 | L4 A1 L17 | A1 L17 bodies 5 in component "inner_adapter"
sketch "Sketch54" plane through (26, 0, 0) normal (-1, 0, 0) x (0, -1, 0)
  line L0 (-183, 125) -> (-38.0516, 125)
  line L1 (-38.0516, 125) -> (-38.0516, 205)
  line L2 (-171.5, 205) -> (-171.5, 133.1623)
  arc A0 (-176.5, 130) -> (-171.5, 133.1623) centre (-173, 130) ccw
  line L3 (-176.5, 130) -> (-176.5, 205)
  line L4 (-105.3085, 180) -> (-105.3085, 170)
  circle A1 centre (-105.3085, 170) radius 1.5
  line L5 (-183, 205) -> (-183, 125)
  line L6 (-176.5, 205) -> (-183, 205)
  line L7 (-38.0516, 205) -> (-171.5, 205)
  dimension "d471" = 10
  dimension "d472" = 3
  constraint coincident L4.end A1.centre
  measures "d471" distance of L4.start L4.end
  measures "d472" diameter of A1
extrude "Extrude24'" cut sketch "Sketch54" against normal blind 5 contours A1 bodies 5 in component "inner_adapter"
extrude "Extrude25" cut sketch "Sketch54" against normal blind 5 from surface at -153 contours A1 bodies 5 in component "inner_adapter"
extrude "Extrude55" add sketch "Sketch92" along normal blind 7 contours L7 L21 L22 L24 L38 | L4 L13 L25 L30 L31 L32 L33 L34 | L6 L9 L25 L27 L28 L29 L30 L34 bodies 5 in component "inner_adapter"
extrude "Extrude56" add sketch "Sketch92" against normal blind 6 contours L7 L21 L22 L24 L38 | L4 L13 L25 L30 L31 L32 L33 L34 | L6 L9 L25 L27 L28 L29 L30 L34 bodies 5 in component "inner_adapter"
extrude "Extrude59" add sketch "Sketch92" along normal blind 1 from surface at -6.5 contours L3 L7 L8 L10 L14 L22 L23 L24 L26 | L7 L21 L22 L24 L38 | L3 L5 L10 L14 L15 L24 L37 L39 | L15 L24 L35 L36 L37 L38 | L3 L6 L8 L9 L10 L14 L23 L26 L29 | L3 L4 L5 L10 L13 L14 L33 L39 | L4 L13 L25 L30 L31 L32 L33 L34 | L6 L9 L25 L27 L28 L29 L30 L34 bodies 5 in component "inner_adapter"
mirror "Mirror9" about plane through (105, 109.0383, 160) normal (-1, 0, 0) of "Extrude55", "Extrude56", "Extrude59" in component "inner_adapter"
sketch "Sketch81" plane through (0, 11, 0) normal (0, -1, 0) x (1, 0, 0)
  line L0 (75, 205) -> (75, 125)
  line L1 (135, 125) -> (135, 205)
  line L2 (105, 132.5) -> (105, 127.5)
  line L3 (105, 133.5) -> (100.0333, 133.5)
  line L4 (100.0333, 133.5) -> (100.0333, 138.5)
  line L5 (100.0333, 138.5) -> (105, 138.5)
  line L6 (105, 138.5) -> (105, 133.5)
  line L7 (105, 138.5) -> (109.9667, 138.5)
  line L8 (109.9667, 138.5) -> (109.9667, 133.5)
  line L9 (109.9667, 133.5) -> (105, 133.5)
  line L10 (105, 133.5) -> (105, 138.5)
  line L11 (105, 130) -> (131, 130)
  line L12 (105, 138.9) -> (110.3667, 138.9)
  line L13 (110.3667, 138.9) -> (110.3667, 133.1)
  line L14 (110.3667, 133.1) -> (105, 133.1)
  line L15 (105, 133.1) -> (99.6333, 133.1)
  line L16 (99.6333, 133.1) -> (99.6333, 138.9)
  line L17 (99.6333, 138.9) -> (105, 138.9)
  line L18 (105, 131.5) -> (98.0333, 131.5)
  line L19 (98.0333, 131.5) -> (98.0333, 140.5)
  line L20 (98.0333, 140.5) -> (105, 140.5)
  line L21 (105, 140.5) -> (111.9667, 140.5)
  line L22 (111.9667, 140.5) -> (111.9667, 131.5)
  line L23 (111.9667, 131.5) -> (105, 131.5)
  line L24 (105, 121.1) -> (110.3667, 121.1)
  line L25 (105, 121.5) -> (109.9667, 121.5)
  line L26 (110.3667, 126.9) -> (105, 126.9)
  line L27 (109.9667, 126.5) -> (105, 126.5)
  line L28 (105, 119.5) -> (111.9667, 119.5)
  line L29 (99.6333, 126.9) -> (99.6333, 121.1)
  line L30 (98.0333, 119.5) -> (105, 119.5)
  line L31 (98.0333, 128.5) -> (98.0333, 119.5)
  line L32 (105, 126.5) -> (100.0333, 126.5)
  line L33 (99.6333, 121.1) -> (105, 121.1)
  line L34 (110.3667, 121.1) -> (110.3667, 126.9)
  line L35 (111.9667, 119.5) -> (111.9667, 128.5)
  line L36 (105, 126.9) -> (99.6333, 126.9)
  line L37 (105, 126.5) -> (105, 121.5)
  line L38 (100.0333, 126.5) -> (100.0333, 121.5)
  line L39 (100.0333, 121.5) -> (105, 121.5)
  line L40 (105, 121.5) -> (105, 126.5)
  line L41 (109.9667, 121.5) -> (109.9667, 126.5)
  line L42 (105, 128.5) -> (98.0333, 128.5)
  line L43 (111.9667, 128.5) -> (105, 128.5)
  line L44 (178.0015, 127.5) -> (32, 127.5)
  line L45 (32, 127.5) -> (32, 132.5)
  line L46 (32, 132.5) -> (178.0015, 132.5)
  line L47 (178.0015, 132.5) -> (178.0015, 127.5)
  line L48 (118, 132.5) -> (118, 127.5)
  line L49 (105, 172) -> (105, 148)
  line L50 (135, 205) -> (75, 205)
  point P0 (105, 127.5)
  dimension "d682" = 5
  dimension "d684" = 5
  dimension "d690" = -0.4
  constraint horizontal L3
  constraint vertical L4
  constraint horizontal L5
  constraint vertical L6
  constraint horizontal L7
  constraint vertical L8
  constraint horizontal L9
  constraint vertical L10
  constraint midpoint L2 L11.start
  constraint perpendicular L2 L11
  constraint symmetric L2.start L11 P0
  constraint symmetric L3.start L11 L27.end
  constraint symmetric L3.end L11 L32.end
  constraint symmetric L4.end L11 L38.end
  constraint symmetric L5.end L11 L25.start
  constraint symmetric L7.end L11 L25.end
  constraint symmetric L8.end L11 L27.start
  constraint symmetric L11 L12.start L24.start
  constraint symmetric L11 L12.end L24.end
  constraint symmetric L11 L13.end L26.start
  constraint symmetric L11 L14.end L26.end
  constraint symmetric L11 L15.end L29.start
  constraint symmetric L11 L16.end L29.end
  constraint symmetric L11 L18.start L42.start
  constraint symmetric L11 L18.end L31.start
  constraint symmetric L11 L19.end L30.start
  constraint symmetric L11 L20.end L28.start
  constraint symmetric L11 L21.end L28.end
  constraint symmetric L11 L22.end L35.end
  constraint coincident L46 L48.start
  constraint coincident L44 L48.end
  constraint perpendicular L44 L48
  constraint horizontal L11
  constraint midpoint L11 L48
  constraint collinear L2 L49
  measures "d682" distance of L3.start L5.end
  measures "d684" distance of L5.end L3.start
extrude "Extrude46" cut sketch "Sketch81" along normal up to surface (-5 mm away) and the other way up to surface (-11 mm away) contours L3 L4 L5 L6 L10 | L6 L7 L8 L9 L10 | L12 L13 L14 L15 L16 L17 | L24 L26 L29 L33 L34 L36 | L25 L27 L37 L40 L41 | L32 L37 L38 L39 L40 bodies 5 in component "inner_adapter"
extrude "Extrude47" add sketch "Sketch81" along normal blind 11 contours L2 L18 L19 L46 | L19 L20 L21 L22 L46 | L28 L30 L31 L35 L44 | L2 L31 L42 L44 | L2 L22 L23 L46 | L2 L35 L43 L44 bodies 5 in component "inner_adapter"
extrude "Extrude48" add 1 faces at (107.3222, 7.3333, 128.5) along direction (0, 0, 1) up to surface (3 mm away) on bodies 5 bodies 5 in component "inner_adapter"
sketch "Sketch82" plane through (0, 11, 0) normal (0, -1, 0) x (1, 0, 0)
  line L0 (111.9667, 125) -> (135, 125)
  line L1 (135, 125) -> (135, 205)
  line L2 (75, 205) -> (75, 125)
  line L3 (137, 124) -> (105, 124)
  line L4 (105, 124) -> (105, 156)
  line L5 (105, 156) -> (137, 156)
  line L6 (137, 156) -> (137, 124)
  line L7 (110.3667, 121.1) -> (99.6333, 121.1)
  line L8 (99.6333, 126.9) -> (110.3667, 126.9)
  line L9 (110.3667, 126.9) -> (110.3667, 121.1)
  line L10 (99.6333, 121.1) -> (99.6333, 126.9)
  line L11 (110.3667, 133.1) -> (99.6333, 133.1)
  line L12 (110.3667, 138.9) -> (110.3667, 133.1)
  line L13 (99.6333, 138.9) -> (110.3667, 138.9)
  line L14 (99.6333, 133.1) -> (99.6333, 138.9)
  line L15 (105, 121.1) -> (105, 124)
  line L16 (99.6333, 136) -> (110.3667, 136)
  line L17 (105, 134) -> (73, 134)
  line L18 (73, 134) -> (73, 168)
  line L19 (73, 168) -> (105, 168)
  line L20 (105, 168) -> (105, 134)
  line L21 (99.6333, 124) -> (110.3667, 124)
  line L22 (99.6333, 136) -> (99.6333, 133.1)
  line L23 (99.6333, 136) -> (99.6334, 134)
  line L24 (111.9667, 140.5) -> (111.9667, 125)
  line L25 (75, 125) -> (98.0333, 125)
  line L26 (98.0333, 125) -> (98.0333, 140.5)
  line L27 (98.0333, 140.5) -> (111.9667, 140.5)
  line L28 (135, 205) -> (75, 205)
  dimension "d696" = 32
  dimension "d697" = 32
  dimension "d699" = 32
  dimension "d700" = 34
  dimension "d752" = 2
  constraint horizontal L3
  constraint vertical L4
  constraint horizontal L5
  constraint vertical L6
  constraint midpoint L7 L15.start
  constraint perpendicular L7 L15
  constraint midpoint L14 L16.start
  constraint midpoint L12 L16.end
  constraint horizontal L17
  constraint vertical L18
  constraint horizontal L19
  constraint vertical L20
  constraint midpoint L10 L21.start
  constraint perpendicular L10 L21
  constraint midpoint L9 L21.end
  constraint coincident L3.end L21
  constraint coincident L3.end L4.start
  constraint collinear L4 L20
  constraint coincident L11.end L14.start
  constraint coincident L17 L23.end
  measures "d696" distance of L3.start L3.end
  measures "d697" distance of L3.start L5.end
  measures "d699" distance of L17.start L17.end
  measures "d700" distance of L17.start L19.end
  measures "d752" distance of L16 L17
extrude "Extrude49" add sketch "Sketch82" along normal blind 11 and the other way blind 1 contours L0 L1 L4 L5 L20 L24 L27 | L0 L1 L3 L4 L5 L6 L8 L9 L11 L12 L13 L20 L24 L27 | L2 L4 L17 L19 L20 L26 L27 | L4 L13 L14 L17 L20 L22 L23 L26 L27 | L2 L17 L18 L19 bodies 5 in component "inner_adapter"